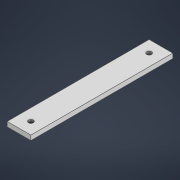
# Autodesk Inventor part: łapa2
Saved by Autodesk Inventor 2022 (Build 260153000, 153)
## iProperties
Created: 2023-04-12
Part Number: łapa2
Material: Ogólny
Document SubType Name: Modeling
Designer: jacek
Density: 1 g/cm^3
Appearance: Domyślna
Author: jacek
Autodesk Inventor part; units mm, degrees
ref_plane "YZ Plane" through (0, 0, 0) normal (1, 0, 0) x (0, 1, 0)
ref_plane "XZ Plane" through (0, 0, 0) normal (0, 1, 0) x (-1, 0, 0)
ref_plane "XY Plane" through (0, 0, 0) normal (0, 0, 1) x (1, 0, 0)
sketch "Szkic1" plane through (0, 0, 0) normal (0, 1, 0) x (-1, 0, 0)
  line L0 (-15, 90) -> (15, 90)
  line L1 (15, 90) -> (15, -90)
  line L2 (15, -90) -> (-15, -90)
  line L3 (-15, -90) -> (-15, 90)
  line L4 (-15, 90) -> (15, -90) construction
  line L5 (15, 90) -> (-15, -90) construction
  point P0 (0, 0)
  dimension "d0" = 30
  dimension "d1" = 180
  constraints: 12 end point, 2 midpoint, 2 parallel, 1 horizontal, 1 perpendicular
  measures "d0" distance of L1.end L2.end
  measures "d1" distance of L0.end L1.end
extrude "Wyciągnięcie proste1" add sketch "Szkic1" along normal blind 6
sketch "Szkic2" plane through (0, 6, 0) normal (0, 1, 0) x (1, 0, 0)
  line L0 (0, 0) -> (0, -75)
  line L1 (0, 0) -> (0, 75)
  dimension "d4" = 75
  dimension "d12" = 75
  constraints: 4 end point, 2 vertical
  measures "d4" distance of L0.start L0.end
  measures "d12" distance of L0.start L1.end
hole "Otwór1" at (0, 6, 75) at (0, 6, -75) direction (0, -1, 0) diameter 6.2 depth 33 tip angle 118
